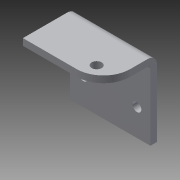
# Autodesk Inventor part: Pneumatic Piston Front Flange (Right Custom)
Saved by Autodesk Inventor 2014 (Build 180170000, 170)
## iProperties
Created: 2014-01-17
Part Number: Pneumatic Piston Front Flange (Right Custom)
Material: Aluminum 6061
Document SubType Name: Sheet Metal
Designer: Michael
Density: 2.71 g/cm^3
Sheet Metal Rule: Default
Appearance: Aluminum - Flat
Author: Michael
Autodesk Inventor part; units mm, degrees
ref_plane "YZ Plane" through (0, 0, 0) normal (1, 0, 0) x (0, 1, 0)
ref_plane "XZ Plane" through (0, 0, 0) normal (0, 1, 0) x (-1, 0, 0)
ref_plane "XY Plane" through (0, 0, 0) normal (0, 0, 1) x (1, 0, 0)
sketch "Sketch1" plane through (0, 0, 0) normal (0, 0, 1) x (1, 0, 0)
  line L0 (0, 0) -> (38.1, 0)
  line L1 (38.1, 0) -> (38.1, 31.75)
  line L2 (38.1, 31.75) -> (0, 31.75)
  line L3 (0, 31.75) -> (0, 0)
  circle A0 centre (6.35, 12.7) radius 2.0701
  line L4 (0, 12.7) -> (38.1, 12.7) construction
  circle A1 centre (31.75, 12.7) radius 2.0701
  dimension "d0" = 38.1
  dimension "d1" = 31.75
  dimension "d2" = 4.1402
  dimension "d3" = 6.35
  dimension "d6" = 25.4
  dimension "d22" = 12.7
  measures "d0" distance of L2.end L1.end
  measures "d1" distance of L1.end L0.end
  measures "d2" diameter of A0
  measures "d3" distance from line of L3 A0.centre
  measures "d6" distance of A0.centre A1.centre
  measures "d22" distance between parallel lines of L0 L4
extrude "Plate1" add sketch "Sketch1" along normal blind 3.175
sketch "Sketch2" plane through (0, 33.02, 4.445) normal (0, 1, 0) x (-1, 0, 0)
  line L0 (-38.1, 0) -> (0, 0)
  line L1 (0, 0) -> (0, 20.955)
  line L2 (0, 20.955) -> (-38.1, 20.955)
  line L3 (-38.1, 20.955) -> (-38.1, 0)
  constraints: 6 end point, 1 horizontal, 1 perpendicular, 1 vertical
edge flange "Flange1" height 25.4 angle 90 thickness 3.175 bend radius 1.27 thickness toward (0, 1, 0) relief straight relief width 3.175 relief depth 1.5875 edges at (19.05, 31.75, 3.175) wall of the first edge with corners at (38.1, 33.02, 4.445) (0, 33.02, 4.445) (0, 33.02, 25.4) (38.1, 33.02, 25.4)
bend "Bend1"
corner "Corner1"
sketch "Sketch4" plane through (0, 36.195, 25.4) normal (0, 1, 0) x (1, 0, 0)
  line L0 (38.1, 0) -> (0, 0) projected
  line L1 (38.1, 20.955) -> (38.1, 0) projected
  circle A0 centre (28.575, 6.35) radius 2.3749
  line L2 (0, 20.955) -> (38.1, 20.955)
  line L3 (38.1, 20.955) -> (38.1, 12.7)
  line L4 (25.4, 0) -> (0, 0)
  line L5 (0, 0) -> (0, 20.955)
  arc A1 (25.4, 0) -> (38.1, 12.7) centre (25.4, 12.7) ccw
  line L6 (25.4, 0) -> (38.1, 0)
  line L7 (38.1, 0) -> (38.1, 12.7)
  point P0 (0, 25.4)
  dimension "d28" = 4.7498
  dimension "d29" = 6.35
  dimension "d30" = 9.525
  dimension "d34" = 12.7
  constraints: 12 end point, 3 tangent, 2 centre point, 2 parallel, 2 point on circle, 2 point on line, 1 collinear, 1 horizontal, 1 perpendicular
  measures "d28" diameter of A0
  measures "d29" distance from line of L0 A0.centre
  measures "d30" distance from line of L1 A0.centre
  measures "d34" radius of A1
extrude "Cut2" cut sketch "Sketch4" against normal blind 3.175 contours L0 A1 L1 | A0
equation "\"d31\" = Thickness"
equation "\"d12\" = BendReliefWidth"
equation "\"d13\" = BendReliefDepth"
equation "\"d14\" = MinimumRemnant"
equation "\"d15\" = BendRadius"
equation "\"d19\" = CornerReliefSize"
equation "\"d20\" = GapSize"
equation "\"d21\" = JacobiRadiusSize"
equation "\"BendRadius\" = Thickness"
equation "\"BendReliefWidth\" = Thickness"
equation "\"BendReliefDepth\" = 0.5 * Thickness"
equation "\"CornerReliefSize\" = 4 * Thickness"
equation "\"MinimumRemnant\" = 2 * Thickness"
equation "\"TransitionRadius\" = BendRadius"
equation "\"JacobiRadiusSize\" = BendRadius"
equation "\"GapSize\" = Thickness"
equation "\"d11\" = BendRadius"
equation "\"Thickness\" = 3.175"
body "Solid1"
